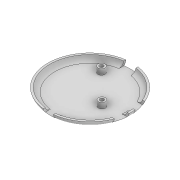
# Autodesk Inventor part: Case top
Saved by Autodesk Inventor 2020 (Build 240168000, 168)
## iProperties
Created: 2022-04-07
Part Number: Case top
Material: Generic
Document SubType Name: Modeling
Designer: ferrerx
Density: 1 g/cm^3
Appearance: Default
Author: ferrerx
Autodesk Inventor part; units mm, degrees
ref_plane "YZ Plane" through (0, 0, 0) normal (1, 0, 0) x (0, 1, 0)
ref_plane "XZ Plane" through (0, 0, 0) normal (0, 1, 0) x (-1, 0, 0)
ref_plane "XY Plane" through (0, 0, 0) normal (0, 0, 1) x (1, 0, 0)
sketch "Sketch1" plane through (0, 0, 0) normal (0, 1, 0) x (-1, 0, 0)
  circle A0 centre (1.143, 0) radius 39 construction
  circle A1 centre (1.143, 0) radius 42
  line L0 (-21.857, 14) -> (-36.857, 14) construction
  line L1 (-36.857, 14) -> (-36.857, 5) construction
  line L2 (-36.857, 5) -> (-21.857, 5) construction
  line L3 (-21.857, 5) -> (-21.857, 14) construction
  line L4 (1.143, 0) -> (-37.857, 0)
  line L5 (0, 0) -> (0, -22) construction
  dimension "d0" = 78
  dimension "d1" = 9
  dimension "d2" = 15
  dimension "d3" = 5
  dimension "d4" = 23
  dimension "d5" = 84
  dimension "d11" = 1.143
  constraints: 12 end point, 2 horizontal, 2 parallel, 1 centre point, 1 coincident, 1 horizontal alignment, 1 perpendicular, 1 point on line, 1 vertical, 3 other
  measures "d1" distance of L0.end L1.end
  measures "d2" distance of L0.start L0.end
  measures "d3" distance from line of point (1.143, 0) L2
  measures "d4" distance from line of point (1.143, 0) L3
  measures "d5" diameter of A1
  measures "d11" distance from line of L5 point (1.143, 0)
extrude "Extrusion1" add sketch "Sketch1" along normal blind 6
fillet "Fillet1" radius 7 1 edges at (40.857, 0, 0)
shell "Shell1" thickness 2 removed faces 1 at (-4.0377, 6, 12.235)
sketch "Sketch2" plane through (-1.143, 2, 0) normal (0, 1, 0) x (1, 0, 0)
  circle A0 centre (-11.303, -22.606) radius 1.95
  circle A1 centre (18.034, 6.223) radius 1.95
  circle A2 centre (-11.303, -22.606) radius 3.5
  circle A3 centre (18.034, 6.223) radius 3.5
  point P0 (1.143, 0)
  dimension "d12" = 3.9
  dimension "d13" = 3.9
  dimension "d14" = 6.223
  dimension "d15" = 16.891
  dimension "d16" = 22.606
  dimension "d17" = 12.446
  dimension "d18" = 7
  dimension "d19" = 7
  constraints: 4 centre point, 2 coincident
  measures "d12" diameter of A0
  measures "d13" diameter of A1
  measures "d14" vertical distance of point (1.143, 0) A1.centre
  measures "d15" horizontal distance of point (1.143, 0) A1.centre
  measures "d16" vertical distance of point (1.143, 0) A0.centre
  measures "d17" horizontal distance of point (1.143, 0) A0.centre
  measures "d18" diameter of A2
  measures "d19" diameter of A3
extrude "Extrusion2" add sketch "Sketch2" along normal blind 5.5
sketch "Sketch3" plane through (-1.143, 2, 0) normal (0, 1, 0) x (1, 0, 0)
  line L0 (7.5, 19.5) -> (-25.5, 19.5) construction
  line L1 (-25.5, 19.5) -> (-25.5, -9.5) construction
  line L2 (-25.5, -9.5) -> (7.5, -9.5) construction
  line L3 (7.5, -9.5) -> (7.5, 19.5) construction
  line L4 (7.5, 19.5) -> (-25.5, -9.5) construction
  line L5 (-25.5, 19.5) -> (7.5, -9.5) construction
  point P0 (1.143, 0)
  point P1 (-9, 5)
  dimension "d22" = 33
  dimension "d23" = 29
  constraints: 12 end point, 2 midpoint, 2 parallel, 1 horizontal, 1 perpendicular
  measures "d22" distance of L0.start L0.end
  measures "d23" distance of L2.end L0.start
sketch "Sketch5" plane through (-1.143, 6, 0) normal (0, 1, 0) x (1, 0, 0)
  line L0 (31.143, -15) -> (45, -15)
  line L1 (45, -15) -> (45, -3)
  line L2 (45, -3) -> (31.143, -3)
  line L3 (31.143, -3) -> (31.143, -15)
  line L4 (1.143, 0) -> (-32, 0) construction
  line L5 (31.143, 15) -> (45, 15)
  line L6 (45, 15) -> (45, 3)
  line L7 (45, 3) -> (31.143, 3)
  line L8 (31.143, 3) -> (31.143, 15)
  line L9 (-5.857, 30) -> (6.143, 30)
  line L10 (6.143, 30) -> (6.143, 46)
  line L11 (6.143, 46) -> (-5.857, 46)
  line L12 (-5.857, 46) -> (-5.857, 30)
  line L13 (-5.857, 30) -> (6.143, 46) construction
  line L14 (6.143, 30) -> (-5.857, 46) construction
  line L15 (-4.873, -22) -> (5.127, -22)
  line L16 (5.127, -22) -> (5.127, -44)
  line L17 (5.127, -44) -> (-4.873, -44)
  line L18 (-4.873, -44) -> (-4.873, -22)
  line L19 (-4.873, -22) -> (5.127, -44) construction
  line L20 (5.127, -22) -> (-4.873, -44) construction
  point P0 (0.143, 38)
  point P1 (0.127, -33)
  dimension "d24" = 3
  dimension "d25" = 12
  dimension "d26" = 30
  dimension "d29" = 1
  dimension "d30" = 12
  dimension "d31" = 1.016
  dimension "d32" = 10
  constraints: 42 end point, 6 parallel, 4 horizontal, 4 midpoint, 4 symmetric about line, 3 perpendicular
  measures "d24" distance from line of L4.start L2
  measures "d25" distance of L0.end L1.end
  measures "d26" distance from line of L4.start L3
  measures "d29" horizontal distance of L4.start point (0.143, 38)
  measures "d30" distance of L10.end L11.end
  measures "d31" horizontal distance of L4.start point (0.127, -33)
  measures "d32" distance of L16.end L17.end
extrude "Extrusion3" cut sketch "Sketch5" against normal up to surface (4 mm away)
mirror "Mirror1" about plane through (0, 0, 0) normal (0, 0, 1) of "Extrusion2"
sketch "Sketch6" plane through (-12.446, 7.5, 22.606) normal (0, 1, 0) x (1, 0, 0)
  circle A0 centre (0, 0) radius 4.9497
  circle A1 centre (29.337, 28.829) radius 1.95 projected
  circle A2 centre (29.337, 28.829) radius 4.3979
  point P0 (12.446, 22.606)
  constraints: 2 centre point, 1 coincident
extrude "Extrusion4" cut sketch "Sketch6" against normal up to surface (5.5 mm away) contours A0 | A1 | A2
body "Solid1"
